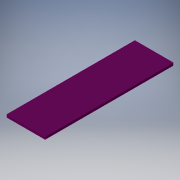
# Autodesk Inventor part: P1001-001-005-320 - Controller Flash
Saved by Autodesk Inventor 2019 (Build 230136000, 136)
## iProperties
Created: 2019-07-16
Part Number: P1001-001-005-320 - Controller Flash
Material: Generic
Document SubType Name: Modeling
Designer: james
Density: 1 g/cm^3
Appearance: Default(1)
Author: james
Autodesk Inventor part; units mm, degrees
ref_plane "YZ Plane" through (0, 0, 0) normal (1, 0, 0) x (0, 1, 0)
ref_plane "XZ Plane" through (0, 0, 0) normal (0, 1, 0) x (-1, 0, 0)
ref_plane "XY Plane" through (0, 0, 0) normal (0, 0, 1) x (1, 0, 0)
sketch "Sketch1" plane through (0, 0, 0) normal (0, 1, 0) x (-1, 0, 0)
  line L0 (7.4219, 46.4844) -> (-22.5781, 46.4844)
  line L1 (-22.5781, 46.4844) -> (-22.5781, -53.5156)
  line L2 (-22.5781, -53.5156) -> (7.4219, -53.5156)
  line L3 (7.4219, -53.5156) -> (7.4219, 46.4844)
  point P0 (0, 0)
  dimension "d0" = 100
  dimension "d1" = 30
  constraints: 8 end point, 2 parallel, 1 horizontal, 1 perpendicular
  measures "d0" distance of L0.end L1.end
  measures "d1" distance of L0.start L0.end
extrude "Extrusion1" add sketch "Sketch1" along normal blind 2
equation "\"d0\" = BoardLength"
equation "\"d1\" = BoardWidth"
equation "\"d2\" = BoardHeight"
equation "\"BoardWidth\" = 30"
equation "\"BoardLength\" = 100"
equation "\"BoardHeight\" = 2"
equation "\"PinsFromEdge\" = 2"
body "Solid1"
